Autodesk Fusion 360 part; units mm, degrees
note: some values were not read from the file. Set by a fixed rule: which sketch regions a step uses.
(part 2 of 6)
sketch "Sketch7" plane through (0, 0, 5.5) normal (0, 0, 1) x (1, 0, 0)
  arc A0 (7.002, -1.8799) -> (7.2083, -0.7765) centre (0, 0) ccw
  line L0 (7.2083, -0.7765) -> (7.9414, -0.8554)
  line L1 (7.9414, -0.8554) -> (7.9421, -0.8555)
  spline S0 degree 5 poles (7.9421, -0.8555) (7.9422, -0.8555) (7.9424, -0.8555) (7.9426, -0.8555) (7.943, -0.8556) (7.9436, -0.8556) (7.9443, -0.8557) (7.945, -0.8557) (7.9458, -0.8558) (7.9468, -0.8559) (7.9478, -0.8559) (7.9489, -0.856) (7.9501, -0.8561) (7.9513, -0.8562) (7.9527, -0.8562) (7.9541, -0.8563) (7.9556, -0.8564) (7.9572, -0.8565) (7.9588, -0.8565) (7.9606, -0.8566) (7.9624, -0.8567) (7.9643, -0.8567) (7.9662, -0.8568) (7.9683, -0.8569) (7.9704, -0.8569) (7.9726, -0.8569) (7.9748, -0.857) (7.9771, -0.857) (7.9795, -0.857) (7.982, -0.8571) (7.9846, -0.8571) (7.9872, -0.8571) (7.9899, -0.8571) (7.9926, -0.8571) (7.9954, -0.857) (7.9983, -0.857) (8.0013, -0.857) (8.0043, -0.8569) (8.0074, -0.8569) (8.0105, -0.8568) (8.0137, -0.8567) (8.017, -0.8566) (8.0203, -0.8565) (8.0237, -0.8564) (8.0272, -0.8563) (8.0307, -0.8561) (8.0343, -0.856) (8.038, -0.8558) (8.0417, -0.8556) (8.0455, -0.8554) (8.0493, -0.8552) (8.0532, -0.855) (8.0571, -0.8547) (8.0611, -0.8545) (8.0652, -0.8542) (8.0693, -0.8539) (8.0735, -0.8536) (8.0777, -0.8533) (8.082, -0.8529) (8.0863, -0.8526) (8.0907, -0.8522) (8.0952, -0.8518) (8.0997, -0.8514) (8.1043, -0.851) (8.1089, -0.8505) (8.1136, -0.8501) (8.1183, -0.8496) (8.123, -0.8491) (8.1279, -0.8486) (8.1327, -0.848) (8.1377, -0.8475) (8.1427, -0.8469) (8.1477, -0.8463) (8.1528, -0.8457) (8.1579, -0.845) (8.1631, -0.8444) (8.1683, -0.8437) (8.1736, -0.843) (8.1789, -0.8422) (8.1842, -0.8415) (8.1897, -0.8407) (8.1951, -0.8399) (8.2006, -0.8391) (8.2062, -0.8383) (8.2118, -0.8374) (8.2174, -0.8365) (8.2231, -0.8356) (8.2289, -0.8347) (8.2346, -0.8338) (8.2405, -0.8328) (8.2463, -0.8318) (8.2523, -0.8308) (8.2582, -0.8297) (8.2642, -0.8287) (8.2703, -0.8276) (8.2763, -0.8264) (8.2825, -0.8253) (8.2886, -0.8241) (8.2948, -0.8229) (8.3011, -0.8217) (8.3074, -0.8205) (8.3137, -0.8192) (8.3201, -0.8179) (8.3265, -0.8166) (8.333, -0.8152) (8.3394, -0.8139) (8.346, -0.8125) (8.3525, -0.8111) (8.3591, -0.8096) (8.3658, -0.8081) (8.3725, -0.8066) (8.3792, -0.8051) (8.386, -0.8035) (8.3927, -0.8019) (8.3996, -0.8003) (8.4064, -0.7987) (8.4134, -0.797) (8.4203, -0.7953) (8.4273, -0.7936) (8.4343, -0.7919) (8.4413, -0.7901) (8.4484, -0.7883) (8.4555, -0.7864) (8.4627, -0.7846) (8.4699, -0.7827) (8.4771, -0.7808) (8.4843, -0.7788) (8.4916, -0.7768) (8.4989, -0.7748) (8.5063, -0.7728) (8.5137, -0.7707) (8.5211, -0.7686) (8.5285, -0.7665) (8.536, -0.7643) (8.5435, -0.7622) (8.5511, -0.7599) (8.5586, -0.7577) (8.5662, -0.7554) (8.5739, -0.7531) (8.5815, -0.7508) (8.5892, -0.7484) (8.597, -0.746) (8.6047, -0.7436) (8.6125, -0.7412) (8.6203, -0.7387) (8.6281, -0.7362) (8.636, -0.7336) (8.6439, -0.7311) (8.6518, -0.7284) (8.6598, -0.7258) (8.6678, -0.7231) (8.6758, -0.7204) (8.6838, -0.7177) (8.6919, -0.7149) (8.7, -0.7122) (8.7081, -0.7093) (8.7163, -0.7065) (8.7244, -0.7036) (8.7326, -0.7007) (8.7408, -0.6977) (8.7491, -0.6947) (8.7574, -0.6917) (8.7657, -0.6887) (8.774, -0.6856) (8.7823, -0.6825) (8.7907, -0.6793) (8.7991, -0.6762) (8.8075, -0.673) (8.816, -0.6697) (8.8245, -0.6665) (8.833, -0.6632) (8.8415, -0.6598) (8.85, -0.6565) (8.8586, -0.6531) (8.8672, -0.6496) (8.8758, -0.6462) (8.8844, -0.6427) (8.8931, -0.6391) (8.9017, -0.6356) (8.9104, -0.632) (8.9191, -0.6283) (8.9279, -0.6247) (8.9366, -0.621) (8.9454, -0.6172) (8.9542, -0.6135) (8.963, -0.6097) (8.9719, -0.6058) (8.9808, -0.602) (8.9896, -0.5981) (8.9985, -0.5942) (9.0075, -0.5902) (9.0164, -0.5862) (9.0254, -0.5822) (9.0343, -0.5781) (9.0433, -0.574) (9.0524, -0.5699) (9.0614, -0.5657) (9.0705, -0.5615) (9.0795, -0.5573) (9.0886, -0.553) (9.0977, -0.5487) (9.1069, -0.5444) (9.116, -0.54) (9.1252, -0.5356) (9.1343, -0.5312) (9.1435, -0.5267) (9.1527, -0.5222) (9.162, -0.5176) (9.1712, -0.5131) (9.1805, -0.5085) (9.1898, -0.5038) (9.199, -0.4991) (9.2084, -0.4944) (9.2177, -0.4897) (9.227, -0.4849) (9.2364, -0.4801) (9.2457, -0.4752) (9.2551, -0.4704) (9.2645, -0.4654) (9.2739, -0.4605) (9.2834, -0.4555) (9.2928, -0.4505) (9.3023, -0.4454) (9.3117, -0.4403) (9.3212, -0.4352) (9.3307, -0.43) (9.3402, -0.4249) (9.3497, -0.4196) (9.3593, -0.4144) (9.3688, -0.4091) (9.3784, -0.4037) (9.3879, -0.3984) (9.3975, -0.3929) (9.4071, -0.3875) (9.4167, -0.382) (9.4264, -0.3765) (9.436, -0.371) (9.4456, -0.3654) (9.4553, -0.3598) (9.465, -0.3541) (9.4746, -0.3485) (9.4824, -0.3439) (9.4882, -0.3404) (9.4921, -0.3381) (9.494, -0.337) knots 0 0 0 0 0 0 0.00416667 0.00833333 0.0125 0.01666667 0.02083333 0.025 0.02916667 0.03333333 0.0375 0.04166667 0.04583333 0.05 0.05416667 0.05833333 0.0625 0.06666667 0.07083333 0.075 0.07916667 0.08333333 0.0875 0.09166667 0.09583333 0.1 0.10416667 0.10833333 0.1125 0.11666667 0.12083333 0.125 0.12916667 0.13333333 0.1375 0.14166667 0.14583333 0.15 0.15416667 0.15833333 0.1625 0.16666667 0.17083333 0.175 0.17916667 0.18333333 0.1875 0.19166667 0.19583333 0.2 0.20416667 0.20833333 0.2125 0.21666667 0.22083333 0.225 0.22916667 0.23333333 0.2375 0.24166667 0.24583333 0.25 0.25416667 0.25833333 0.2625 0.26666667 0.27083333 0.275 0.27916667 0.28333333 0.2875 0.29166667 0.29583333 0.3 0.30416667 0.30833333 0.3125 0.31666667 0.32083333 0.325 0.32916667 0.33333333 0.3375 0.34166667 0.34583333 0.35 0.35416667 0.35833333 0.3625 0.36666667 0.37083333 0.375 0.37916667 0.38333333 0.3875 0.39166667 0.39583333 0.4 0.40416667 0.40833333 0.4125 0.41666667 0.42083333 0.425 0.42916667 0.43333333 0.4375 0.44166667 0.44583333 0.45 0.45416667 0.45833333 0.4625 0.46666667 0.47083333 0.475 0.47916667 0.48333333 0.4875 0.49166667 0.49583333 0.5 0.50416667 0.50833333 0.5125 0.51666667 0.52083333 0.525 0.52916667 0.53333333 0.5375 0.54166667 0.54583333 0.55 0.55416667 0.55833333 0.5625 0.56666667 0.57083333 0.575 0.57916667 0.58333333 0.5875 0.59166667 0.59583333 0.6 0.60416667 0.60833333 0.6125 0.61666667 0.62083333 0.625 0.62916667 0.63333333 0.6375 0.64166667 0.64583333 0.65 0.65416667 0.65833333 0.6625 0.66666667 0.67083333 0.675 0.67916667 0.68333333 0.6875 0.69166667 0.69583333 0.7 0.70416667 0.70833333 0.7125 0.71666667 0.72083333 0.725 0.72916667 0.73333333 0.7375 0.74166667 0.74583333 0.75 0.75416667 0.75833333 0.7625 0.76666667 0.77083333 0.775 0.77916667 0.78333333 0.7875 0.79166667 0.79583333 0.8 0.80416667 0.80833333 0.8125 0.81666667 0.82083333 0.825 0.82916667 0.83333333 0.8375 0.84166667 0.84583333 0.85 0.85416667 0.85833333 0.8625 0.86666667 0.87083333 0.875 0.87916667 0.88333333 0.8875 0.89166667 0.89583333 0.9 0.90416667 0.90833333 0.9125 0.91666667 0.92083333 0.925 0.92916667 0.93333333 0.9375 0.94166667 0.94583333 0.95 0.95416667 0.95833333 0.9625 0.96666667 0.97083333 0.975 0.97916667 0.98333333 0.9875 0.99166667 0.99583333 1 1 1 1 1 1
  arc A1 (9.494, -0.337) -> (9.494, 0.337) centre (0, 0) ccw
  spline S1 degree 5 poles (9.494, 0.337) (9.4921, 0.3381) (9.4882, 0.3404) (9.4824, 0.3439) (9.4746, 0.3485) (9.465, 0.3541) (9.4553, 0.3598) (9.4456, 0.3654) (9.436, 0.371) (9.4264, 0.3765) (9.4167, 0.382) (9.4071, 0.3875) (9.3975, 0.3929) (9.3879, 0.3984) (9.3784, 0.4037) (9.3688, 0.4091) (9.3593, 0.4144) (9.3497, 0.4196) (9.3402, 0.4249) (9.3307, 0.43) (9.3212, 0.4352) (9.3117, 0.4403) (9.3023, 0.4454) (9.2928, 0.4505) (9.2834, 0.4555) (9.2739, 0.4605) (9.2645, 0.4654) (9.2551, 0.4704) (9.2457, 0.4752) (9.2364, 0.4801) (9.227, 0.4849) (9.2177, 0.4897) (9.2084, 0.4944) (9.199, 0.4991) (9.1898, 0.5038) (9.1805, 0.5085) (9.1712, 0.5131) (9.162, 0.5176) (9.1527, 0.5222) (9.1435, 0.5267) (9.1343, 0.5312) (9.1252, 0.5356) (9.116, 0.54) (9.1069, 0.5444) (9.0977, 0.5487) (9.0886, 0.553) (9.0795, 0.5573) (9.0705, 0.5615) (9.0614, 0.5657) (9.0524, 0.5699) (9.0433, 0.574) (9.0343, 0.5781) (9.0254, 0.5822) (9.0164, 0.5862) (9.0075, 0.5902) (8.9985, 0.5942) (8.9896, 0.5981) (8.9808, 0.602) (8.9719, 0.6058) (8.963, 0.6097) (8.9542, 0.6135) (8.9454, 0.6172) (8.9366, 0.621) (8.9279, 0.6247) (8.9191, 0.6283) (8.9104, 0.632) (8.9017, 0.6356) (8.8931, 0.6391) (8.8844, 0.6427) (8.8758, 0.6462) (8.8672, 0.6496) (8.8586, 0.6531) (8.85, 0.6565) (8.8415, 0.6598) (8.833, 0.6632) (8.8245, 0.6665) (8.816, 0.6697) (8.8075, 0.673) (8.7991, 0.6762) (8.7907, 0.6793) (8.7823, 0.6825) (8.774, 0.6856) (8.7657, 0.6887) (8.7574, 0.6917) (8.7491, 0.6947) (8.7408, 0.6977) (8.7326, 0.7007) (8.7244, 0.7036) (8.7163, 0.7065) (8.7081, 0.7093) (8.7, 0.7122) (8.6919, 0.7149) (8.6838, 0.7177) (8.6758, 0.7204) (8.6678, 0.7231) (8.6598, 0.7258) (8.6518, 0.7284) (8.6439, 0.7311) (8.636, 0.7336) (8.6281, 0.7362) (8.6203, 0.7387) (8.6125, 0.7412) (8.6047, 0.7436) (8.597, 0.746) (8.5892, 0.7484) (8.5815, 0.7508) (8.5739, 0.7531) (8.5662, 0.7554) (8.5586, 0.7577) (8.5511, 0.7599) (8.5435, 0.7622) (8.536, 0.7643) (8.5285, 0.7665) (8.5211, 0.7686) (8.5137, 0.7707) (8.5063, 0.7728) (8.4989, 0.7748) (8.4916, 0.7768) (8.4843, 0.7788) (8.4771, 0.7808) (8.4699, 0.7827) (8.4627, 0.7846) (8.4555, 0.7864) (8.4484, 0.7883) (8.4413, 0.7901) (8.4343, 0.7919) (8.4273, 0.7936) (8.4203, 0.7953) (8.4134, 0.797) (8.4064, 0.7987) (8.3996, 0.8003) (8.3927, 0.8019) (8.386, 0.8035) (8.3792, 0.8051) (8.3725, 0.8066) (8.3658, 0.8081) (8.3591, 0.8096) (8.3525, 0.8111) (8.346, 0.8125) (8.3394, 0.8139) (8.333, 0.8152) (8.3265, 0.8166) (8.3201, 0.8179) (8.3137, 0.8192) (8.3074, 0.8205) (8.3011, 0.8217) (8.2948, 0.8229) (8.2886, 0.8241) (8.2825, 0.8253) (8.2763, 0.8264) (8.2703, 0.8276) (8.2642, 0.8287) (8.2582, 0.8297) (8.2523, 0.8308) (8.2463, 0.8318) (8.2405, 0.8328) (8.2346, 0.8338) (8.2289, 0.8347) (8.2231, 0.8356) (8.2174, 0.8365) (8.2118, 0.8374) (8.2062, 0.8383) (8.2006, 0.8391) (8.1951, 0.8399) (8.1897, 0.8407) (8.1842, 0.8415) (8.1789, 0.8422) (8.1736, 0.843) (8.1683, 0.8437) (8.1631, 0.8444) (8.1579, 0.845) (8.1528, 0.8457) (8.1477, 0.8463) (8.1427, 0.8469) (8.1377, 0.8475) (8.1327, 0.848) (8.1279, 0.8486) (8.123, 0.8491) (8.1183, 0.8496) (8.1136, 0.8501) (8.1089, 0.8505) (8.1043, 0.851) (8.0997, 0.8514) (8.0952, 0.8518) (8.0907, 0.8522) (8.0863, 0.8526) (8.082, 0.8529) (8.0777, 0.8533) (8.0735, 0.8536) (8.0693, 0.8539) (8.0652, 0.8542) (8.0611, 0.8545) (8.0571, 0.8547) (8.0532, 0.855) (8.0493, 0.8552) (8.0455, 0.8554) (8.0417, 0.8556) (8.038, 0.8558) (8.0343, 0.856) (8.0307, 0.8561) (8.0272, 0.8563) (8.0237, 0.8564) (8.0203, 0.8565) (8.017, 0.8566) (8.0137, 0.8567) (8.0105, 0.8568) (8.0074, 0.8569) (8.0043, 0.8569) (8.0013, 0.857) (7.9983, 0.857) (7.9954, 0.857) (7.9926, 0.8571) (7.9899, 0.8571) (7.9872, 0.8571) (7.9846, 0.8571) (7.982, 0.8571) (7.9795, 0.857) (7.9771, 0.857) (7.9748, 0.857) (7.9726, 0.8569) (7.9704, 0.8569) (7.9683, 0.8569) (7.9662, 0.8568) (7.9643, 0.8567) (7.9624, 0.8567) (7.9606, 0.8566) (7.9588, 0.8565) (7.9572, 0.8565) (7.9556, 0.8564) (7.9541, 0.8563) (7.9527, 0.8562) (7.9513, 0.8562) (7.9501, 0.8561) (7.9489, 0.856) (7.9478, 0.8559) (7.9468, 0.8559) (7.9458, 0.8558) (7.945, 0.8557) (7.9443, 0.8557) (7.9436, 0.8556) (7.943, 0.8556) (7.9426, 0.8555) (7.9424, 0.8555) (7.9422, 0.8555) (7.9421, 0.8555) knots -1 -1 -1 -1 -1 -1 -0.99583333 -0.99166667 -0.9875 -0.98333333 -0.97916667 -0.975 -0.97083333 -0.96666667 -0.9625 -0.95833333 -0.95416667 -0.95 -0.94583333 -0.94166667 -0.9375 -0.93333333 -0.92916667 -0.925 -0.92083333 -0.91666667 -0.9125 -0.90833333 -0.90416667 -0.9 -0.89583333 -0.89166667 -0.8875 -0.88333333 -0.87916667 -0.875 -0.87083333 -0.86666667 -0.8625 -0.85833333 -0.85416667 -0.85 -0.84583333 -0.84166667 -0.8375 -0.83333333 -0.82916667 -0.825 -0.82083333 -0.81666667 -0.8125 -0.80833333 -0.80416667 -0.8 -0.79583333 -0.79166667 -0.7875 -0.78333333 -0.77916667 -0.775 -0.77083333 -0.76666667 -0.7625 -0.75833333 -0.75416667 -0.75 -0.74583333 -0.74166667 -0.7375 -0.73333333 -0.72916667 -0.725 -0.72083333 -0.71666667 -0.7125 -0.70833333 -0.70416667 -0.7 -0.69583333 -0.69166667 -0.6875 -0.68333333 -0.67916667 -0.675 -0.67083333 -0.66666667 -0.6625 -0.65833333 -0.65416667 -0.65 -0.64583333 -0.64166667 -0.6375 -0.63333333 -0.62916667 -0.625 -0.62083333 -0.61666667 -0.6125 -0.60833333 -0.60416667 -0.6 -0.59583333 -0.59166667 -0.5875 -0.58333333 -0.57916667 -0.575 -0.57083333 -0.56666667 -0.5625 -0.55833333 -0.55416667 -0.55 -0.54583333 -0.54166667 -0.5375 -0.53333333 -0.52916667 -0.525 -0.52083333 -0.51666667 -0.5125 -0.50833333 -0.50416667 -0.5 -0.49583333 -0.49166667 -0.4875 -0.48333333 -0.47916667 -0.475 -0.47083333 -0.46666667 -0.4625 -0.45833333 -0.45416667 -0.45 -0.44583333 -0.44166667 -0.4375 -0.43333333 -0.42916667 -0.425 -0.42083333 -0.41666667 -0.4125 -0.40833333 -0.40416667 -0.4 -0.39583333 -0.39166667 -0.3875 -0.38333333 -0.37916667 -0.375 -0.37083333 -0.36666667 -0.3625 -0.35833333 -0.35416667 -0.35 -0.34583333 -0.34166667 -0.3375 -0.33333333 -0.32916667 -0.325 -0.32083333 -0.31666667 -0.3125 -0.30833333 -0.30416667 -0.3 -0.29583333 -0.29166667 -0.2875 -0.28333333 -0.27916667 -0.275 -0.27083333 -0.26666667 -0.2625 -0.25833333 -0.25416667 -0.25 -0.24583333 -0.24166667 -0.2375 -0.23333333 -0.22916667 -0.225 -0.22083333 -0.21666667 -0.2125 -0.20833333 -0.20416667 -0.2 -0.19583333 -0.19166667 -0.1875 -0.18333333 -0.17916667 -0.175 -0.17083333 -0.16666667 -0.1625 -0.15833333 -0.15416667 -0.15 -0.14583333 -0.14166667 -0.1375 -0.13333333 -0.12916667 -0.125 -0.12083333 -0.11666667 -0.1125 -0.10833333 -0.10416667 -0.1 -0.09583333 -0.09166667 -0.0875 -0.08333333 -0.07916667 -0.075 -0.07083333 -0.06666667 -0.0625 -0.05833333 -0.05416667 -0.05 -0.04583333 -0.04166667 -0.0375 -0.03333333 -0.02916667 -0.025 -0.02083333 -0.01666667 -0.0125 -0.00833333 -0.00416667 0 0 0 0 0 0
  line L2 (7.9421, 0.8555) -> (7.9414, 0.8554)
  line L3 (7.9414, 0.8554) -> (7.2083, 0.7765)
  arc A2 (7.2083, 0.7765) -> (7.002, 1.8799) centre (0, 0) ccw
  line L4 (7.002, 1.8799) -> (7.7142, 2.0711)
  line L5 (7.7142, 2.0711) -> (7.7149, 2.0713)
  spline S2 degree 5 poles (7.7149, 2.0713) (7.7149, 2.0713) (7.7151, 2.0714) (7.7153, 2.0714) (7.7157, 2.0715) (7.7163, 2.0717) (7.7169, 2.0719) (7.7176, 2.0721) (7.7184, 2.0723) (7.7193, 2.0726) (7.7203, 2.0729) (7.7213, 2.0732) (7.7225, 2.0736) (7.7237, 2.074) (7.7249, 2.0744) (7.7263, 2.0749) (7.7277, 2.0753) (7.7292, 2.0758) (7.7308, 2.0764) (7.7324, 2.0769) (7.7342, 2.0775) (7.7359, 2.0781) (7.7378, 2.0788) (7.7397, 2.0795) (7.7417, 2.0802) (7.7438, 2.0809) (7.7459, 2.0817) (7.7481, 2.0825) (7.7503, 2.0834) (7.7526, 2.0842) (7.755, 2.0852) (7.7574, 2.0861) (7.7599, 2.0871) (7.7625, 2.0881) (7.7651, 2.0891) (7.7678, 2.0902) (7.7705, 2.0913) (7.7733, 2.0924) (7.7762, 2.0936) (7.7791, 2.0948) (7.7821, 2.096) (7.7851, 2.0973) (7.7882, 2.0986) (7.7913, 2.0999) (7.7945, 2.1013) (7.7977, 2.1027) (7.801, 2.1042) (7.8043, 2.1057) (7.8077, 2.1072) (7.8112, 2.1087) (7.8147, 2.1103) (7.8182, 2.1119) (7.8218, 2.1136) (7.8254, 2.1153) (7.8291, 2.117) (7.8329, 2.1187) (7.8367, 2.1205) (7.8405, 2.1224) (7.8444, 2.1242) (7.8483, 2.1261) (7.8522, 2.1281) (7.8563, 2.13) (7.8603, 2.132) (7.8644, 2.1341) (7.8686, 2.1362) (7.8727, 2.1383) (7.877, 2.1404) (7.8812, 2.1426) (7.8856, 2.1449) (7.8899, 2.1471) (7.8943, 2.1494) (7.8987, 2.1518) (7.9032, 2.1541) (7.9077, 2.1566) (7.9123, 2.159) (7.9168, 2.1615) (7.9215, 2.164) (7.9261, 2.1666) (7.9308, 2.1692) (7.9356, 2.1718) (7.9403, 2.1745) (7.9451, 2.1772) (7.95, 2.18) (7.9549, 2.1827) (7.9598, 2.1856) (7.9647, 2.1884) (7.9697, 2.1913) (7.9747, 2.1943) (7.9798, 2.1972) (7.9849, 2.2002) (7.99, 2.2033) (7.9951, 2.2064) (8.0003, 2.2095) (8.0055, 2.2127) (8.0107, 2.2159) (8.016, 2.2191) (8.0213, 2.2224) (8.0266, 2.2257) (8.032, 2.2291) (8.0374, 2.2325) (8.0428, 2.2359) (8.0482, 2.2394) (8.0537, 2.2429) (8.0592, 2.2464) (8.0647, 2.25) (8.0703, 2.2536) (8.0759, 2.2573) (8.0815, 2.261) (8.0871, 2.2647) (8.0928, 2.2685) (8.0985, 2.2723) (8.1042, 2.2762) (8.1099, 2.2801) (8.1157, 2.284) (8.1215, 2.288) (8.1273, 2.292) (8.1331, 2.2961) (8.139, 2.3001) (8.1449, 2.3043) (8.1508, 2.3084) (8.1567, 2.3126) (8.1627, 2.3169) (8.1686, 2.3212) (8.1746, 2.3255) (8.1806, 2.3298) (8.1867, 2.3342) (8.1927, 2.3387) (8.1988, 2.3432) (8.2049, 2.3477) (8.211, 2.3522) (8.2172, 2.3568) (8.2233, 2.3614) (8.2295, 2.3661) (8.2357, 2.3708) (8.2419, 2.3756) (8.2481, 2.3804) (8.2544, 2.3852) (8.2607, 2.3901) (8.267, 2.395) (8.2733, 2.3999) (8.2796, 2.4049) (8.2859, 2.4099) (8.2923, 2.415) (8.2986, 2.4201) (8.305, 2.4252) (8.3114, 2.4304) (8.3179, 2.4356) (8.3243, 2.4409) (8.3307, 2.4462) (8.3372, 2.4515) (8.3437, 2.4569) (8.3502, 2.4623) (8.3567, 2.4677) (8.3632, 2.4732) (8.3698, 2.4787) (8.3763, 2.4843) (8.3829, 2.4899) (8.3895, 2.4955) (8.396, 2.5012) (8.4026, 2.507) (8.4093, 2.5127) (8.4159, 2.5185) (8.4225, 2.5244) (8.4292, 2.5302) (8.4358, 2.5361) (8.4425, 2.5421) (8.4492, 2.5481) (8.4559, 2.5541) (8.4626, 2.5602) (8.4693, 2.5663) (8.476, 2.5725) (8.4828, 2.5786) (8.4895, 2.5849) (8.4963, 2.5911) (8.503, 2.5974) (8.5098, 2.6038) (8.5166, 2.6102) (8.5234, 2.6166) (8.5302, 2.623) (8.537, 2.6295) (8.5438, 2.6361) (8.5507, 2.6426) (8.5575, 2.6493) (8.5643, 2.6559) (8.5712, 2.6626) (8.578, 2.6693) (8.5849, 2.6761) (8.5918, 2.6829) (8.5986, 2.6897) (8.6055, 2.6966) (8.6124, 2.7035) (8.6193, 2.7105) (8.6262, 2.7175) (8.6331, 2.7245) (8.64, 2.7316) (8.6469, 2.7387) (8.6539, 2.7459) (8.6608, 2.753) (8.6677, 2.7603) (8.6747, 2.7675) (8.6816, 2.7748) (8.6885, 2.7822) (8.6955, 2.7895) (8.7024, 2.797) (8.7094, 2.8044) (8.7164, 2.8119) (8.7233, 2.8194) (8.7303, 2.827) (8.7372, 2.8346) (8.7442, 2.8422) (8.7512, 2.8499) (8.7582, 2.8576) (8.7651, 2.8654) (8.7721, 2.8732) (8.7791, 2.881) (8.7861, 2.8889) (8.7931, 2.8968) (8.8001, 2.9047) (8.807, 2.9127) (8.814, 2.9207) (8.821, 2.9288) (8.828, 2.9369) (8.835, 2.945) (8.842, 2.9532) (8.849, 2.9614) (8.856, 2.9696) (8.863, 2.9779) (8.8699, 2.9862) (8.8769, 2.9946) (8.8839, 3.003) (8.8909, 3.0114) (8.8979, 3.0199) (8.9049, 3.0284) (8.9119, 3.0369) (8.9189, 3.0455) (8.9258, 3.0541) (8.9328, 3.0627) (8.9398, 3.0714) (8.9468, 3.0802) (8.9537, 3.0889) (8.9607, 3.0977) (8.9663, 3.1048) (8.9705, 3.1101) (8.9732, 3.1136) (8.9746, 3.1154) knots 0 0 0 0 0 0 0.00416667 0.00833333 0.0125 0.01666667 0.02083333 0.025 0.02916667 0.03333333 0.0375 0.04166667 0.04583333 0.05 0.05416667 0.05833333 0.0625 0.06666667 0.07083333 0.075 0.07916667 0.08333333 0.0875 0.09166667 0.09583333 0.1 0.10416667 0.10833333 0.1125 0.11666667 0.12083333 0.125 0.12916667 0.13333333 0.1375 0.14166667 0.14583333 0.15 0.15416667 0.15833333 0.1625 0.16666667 0.17083333 0.175 0.17916667 0.18333333 0.1875 0.19166667 0.19583333 0.2 0.20416667 0.20833333 0.2125 0.21666667 0.22083333 0.225 0.22916667 0.23333333 0.2375 0.24166667 0.24583333 0.25 0.25416667 0.25833333 0.2625 0.26666667 0.27083333 0.275 0.27916667 0.28333333 0.2875 0.29166667 0.29583333 0.3 0.30416667 0.30833333 0.3125 0.31666667 0.32083333 0.325 0.32916667 0.33333333 0.3375 0.34166667 0.34583333 0.35 0.35416667 0.35833333 0.3625 0.36666667 0.37083333 0.375 0.37916667 0.38333333 0.3875 0.39166667 0.39583333 0.4 0.40416667 0.40833333 0.4125 0.41666667 0.42083333 0.425 0.42916667 0.43333333 0.4375 0.44166667 0.44583333 0.45 0.45416667 0.45833333 0.4625 0.46666667 0.47083333 0.475 0.47916667 0.48333333 0.4875 0.49166667 0.49583333 0.5 0.50416667 0.50833333 0.5125 0.51666667 0.52083333 0.525 0.52916667 0.53333333 0.5375 0.54166667 0.54583333 0.55 0.55416667 0.55833333 0.5625 0.56666667 0.57083333 0.575 0.57916667 0.58333333 0.5875 0.59166667 0.59583333 0.6 0.60416667 0.60833333 0.6125 0.61666667 0.62083333 0.625 0.62916667 0.63333333 0.6375 0.64166667 0.64583333 0.65 0.65416667 0.65833333 0.6625 0.66666667 0.67083333 0.675 0.67916667 0.68333333 0.6875 0.69166667 0.69583333 0.7 0.70416667 0.70833333 0.7125 0.71666667 0.72083333 0.725 0.72916667 0.73333333 0.7375 0.74166667 0.74583333 0.75 0.75416667 0.75833333 0.7625 0.76666667 0.77083333 0.775 0.77916667 0.78333333 0.7875 0.79166667 0.79583333 0.8 0.80416667 0.80833333 0.8125 0.81666667 0.82083333 0.825 0.82916667 0.83333333 0.8375 0.84166667 0.84583333 0.85 0.85416667 0.85833333 0.8625 0.86666667 0.87083333 0.875 0.87916667 0.88333333 0.8875 0.89166667 0.89583333 0.9 0.90416667 0.90833333 0.9125 0.91666667 0.92083333 0.925 0.92916667 0.93333333 0.9375 0.94166667 0.94583333 0.95 0.95416667 0.95833333 0.9625 0.96666667 0.97083333 0.975 0.97916667 0.98333333 0.9875 0.99166667 0.99583333 1 1 1 1 1 1
  arc A3 (8.9746, 3.1154) -> (8.7312, 3.7439) centre (0, 0) ccw
  spline S3 degree 5 poles (8.7312, 3.7439) (8.729, 3.7442) (8.7245, 3.745) (8.7178, 3.7461) (8.709, 3.7476) (8.6979, 3.7494) (8.6868, 3.7511) (8.6758, 3.7529) (8.6648, 3.7546) (8.6538, 3.7563) (8.6428, 3.758) (8.6319, 3.7596) (8.621, 3.7612) (8.6101, 3.7628) (8.5992, 3.7643) (8.5884, 3.7658) (8.5776, 3.7673) (8.5668, 3.7688) (8.556, 3.7702) (8.5453, 3.7716) (8.5345, 3.773) (8.5239, 3.7744) (8.5132, 3.7757) (8.5025, 3.777) (8.4919, 3.7783) (8.4813, 3.7795) (8.4708, 3.7807) (8.4602, 3.7819) (8.4497, 3.7831) (8.4392, 3.7842) (8.4288, 3.7853) (8.4183, 3.7864) (8.4079, 3.7875) (8.3975, 3.7885) (8.3872, 3.7895) (8.3769, 3.7905) (8.3666, 3.7915) (8.3563, 3.7924) (8.346, 3.7933) (8.3358, 3.7941) (8.3256, 3.795) (8.3155, 3.7958) (8.3053, 3.7966) (8.2952, 3.7974) (8.2852, 3.7981) (8.2751, 3.7989) (8.2651, 3.7995) (8.2551, 3.8002) (8.2451, 3.8009) (8.2352, 3.8015) (8.2253, 3.8021) (8.2154, 3.8026) (8.2056, 3.8032) (8.1958, 3.8037) (8.186, 3.8042) (8.1763, 3.8047) (8.1665, 3.8051) (8.1568, 3.8056) (8.1472, 3.806) (8.1376, 3.8063) (8.128, 3.8067) (8.1184, 3.807) (8.1089, 3.8073) (8.0993, 3.8076) (8.0899, 3.8079) (8.0804, 3.8081) (8.071, 3.8083) (8.0616, 3.8085) (8.0523, 3.8087) (8.043, 3.8088) (8.0337, 3.8089) (8.0245, 3.809) (8.0153, 3.8091) (8.0061, 3.8092) (7.9969, 3.8092) (7.9878, 3.8092) (7.9787, 3.8092) (7.9697, 3.8092) (7.9607, 3.8091) (7.9517, 3.809) (7.9428, 3.809) (7.9338, 3.8088) (7.925, 3.8087) (7.9161, 3.8085) (7.9073, 3.8084) (7.8986, 3.8082) (7.8898, 3.8079) (7.8811, 3.8077) (7.8725, 3.8074) (7.8638, 3.8072) (7.8552, 3.8069) (7.8467, 3.8065) (7.8382, 3.8062) (7.8297, 3.8058) (7.8212, 3.8055) (7.8128, 3.8051) (7.8045, 3.8047) (7.7961, 3.8042) (7.7878, 3.8038) (7.7796, 3.8033) (7.7713, 3.8028) (7.7632, 3.8023) (7.755, 3.8018) (7.7469, 3.8012) (7.7388, 3.8007) (7.7308, 3.8001) (7.7228, 3.7995) (7.7149, 3.7989) (7.707, 3.7983) (7.6991, 3.7976) (7.6913, 3.797) (7.6835, 3.7963) (7.6757, 3.7956) (7.668, 3.7949) (7.6603, 3.7942) (7.6527, 3.7934) (7.6451, 3.7927) (7.6376, 3.7919) (7.6301, 3.7911) (7.6226, 3.7903) (7.6152, 3.7895) (7.6078, 3.7887) (7.6004, 3.7878) (7.5931, 3.787) (7.5859, 3.7861) (7.5787, 3.7852) (7.5715, 3.7843) (7.5644, 3.7834) (7.5573, 3.7825) (7.5503, 3.7815) (7.5433, 3.7806) (7.5363, 3.7796) (7.5294, 3.7786) (7.5225, 3.7776) (7.5157, 3.7766) (7.5089, 3.7756) (7.5022, 3.7746) (7.4955, 3.7736) (7.4889, 3.7725) (7.4823, 3.7715) (7.4757, 3.7704) (7.4692, 3.7693) (7.4628, 3.7682) (7.4564, 3.7672) (7.45, 3.766) (7.4437, 3.7649) (7.4374, 3.7638) (7.4312, 3.7627) (7.425, 3.7615) (7.4189, 3.7604) (7.4128, 3.7592) (7.4068, 3.7581) (7.4008, 3.7569) (7.3949, 3.7557) (7.389, 3.7545) (7.3832, 3.7534) (7.3774, 3.7522) (7.3717, 3.751) (7.366, 3.7498) (7.3603, 3.7485) (7.3548, 3.7473) (7.3492, 3.7461) (7.3437, 3.7449) (7.3383, 3.7436) (7.3329, 3.7424) (7.3276, 3.7412) (7.3223, 3.7399) (7.3171, 3.7387) (7.3119, 3.7374) (7.3068, 3.7362) (7.3017, 3.7349) (7.2967, 3.7337) (7.2918, 3.7324) (7.2869, 3.7312) (7.282, 3.7299) (7.2772, 3.7286) (7.2725, 3.7274) (7.2678, 3.7261) (7.2632, 3.7249) (7.2586, 3.7236) (7.2541, 3.7224) (7.2496, 3.7211) (7.2452, 3.7199) (7.2408, 3.7186) (7.2365, 3.7174) (7.2323, 3.7161) (7.2281, 3.7149) (7.224, 3.7137) (7.2199, 3.7124) (7.2159, 3.7112) (7.212, 3.71) (7.2081, 3.7088) (7.2043, 3.7076) (7.2005, 3.7064) (7.1968, 3.7052) (7.1932, 3.704) (7.1896, 3.7028) (7.186, 3.7016) (7.1826, 3.7005) (7.1792, 3.6993) (7.1758, 3.6982) (7.1726, 3.6971) (7.1693, 3.696) (7.1662, 3.6948) (7.1631, 3.6937) (7.1601, 3.6927) (7.1571, 3.6916) (7.1542, 3.6905) (7.1514, 3.6895) (7.1486, 3.6885) (7.1459, 3.6875) (7.1433, 3.6865) (7.1407, 3.6855) (7.1382, 3.6845) (7.1358, 3.6836) (7.1334, 3.6826) (7.1311, 3.6817) (7.1289, 3.6808) (7.1267, 3.6799) (7.1246, 3.6791) (7.1226, 3.6783) (7.1206, 3.6775) (7.1188, 3.6767) (7.117, 3.6759) (7.1152, 3.6752) (7.1136, 3.6744) (7.112, 3.6738) (7.1104, 3.6731) (7.109, 3.6725) (7.1076, 3.6718) (7.1063, 3.6713) (7.1051, 3.6707) (7.104, 3.6702) (7.1029, 3.6697) (7.1019, 3.6692) (7.101, 3.6688) (7.1001, 3.6684) (7.0994, 3.668) (7.0987, 3.6677) (7.0981, 3.6674) (7.0976, 3.6672) (7.0972, 3.667) (7.097, 3.6669) (7.0968, 3.6668) (7.0968, 3.6668) knots -1 -1 -1 -1 -1 -1 -0.99583333 -0.99166667 -0.9875 -0.98333333 -0.97916667 -0.975 -0.97083333 -0.96666667 -0.9625 -0.95833333 -0.95416667 -0.95 -0.94583333 -0.94166667 -0.9375 -0.93333333 -0.92916667 -0.925 -0.92083333 -0.91666667 -0.9125 -0.90833333 -0.90416667 -0.9 -0.89583333 -0.89166667 -0.8875 -0.88333333 -0.87916667 -0.875 -0.87083333 -0.86666667 -0.8625 -0.85833333 -0.85416667 -0.85 -0.84583333 -0.84166667 -0.8375 -0.83333333 -0.82916667 -0.825 -0.82083333 -0.81666667 -0.8125 -0.80833333 -0.80416667 -0.8 -0.79583333 -0.79166667 -0.7875 -0.78333333 -0.77916667 -0.775 -0.77083333 -0.76666667 -0.7625 -0.75833333 -0.75416667 -0.75 -0.74583333 -0.74166667 -0.7375 -0.73333333 -0.72916667 -0.725 -0.72083333 -0.71666667 -0.7125 -0.70833333 -0.70416667 -0.7 -0.69583333 -0.69166667 -0.6875 -0.68333333 -0.67916667 -0.675 -0.67083333 -0.66666667 -0.6625 -0.65833333 -0.65416667 -0.65 -0.64583333 -0.64166667 -0.6375 -0.63333333 -0.62916667 -0.625 -0.62083333 -0.61666667 -0.6125 -0.60833333 -0.60416667 -0.6 -0.59583333 -0.59166667 -0.5875 -0.58333333 -0.57916667 -0.575 -0.57083333 -0.56666667 -0.5625 -0.55833333 -0.55416667 -0.55 -0.54583333 -0.54166667 -0.5375 -0.53333333 -0.52916667 -0.525 -0.52083333 -0.51666667 -0.5125 -0.50833333 -0.50416667 -0.5 -0.49583333 -0.49166667 -0.4875 -0.48333333 -0.47916667 -0.475 -0.47083333 -0.46666667 -0.4625 -0.45833333 -0.45416667 -0.45 -0.44583333 -0.44166667 -0.4375 -0.43333333 -0.42916667 -0.425 -0.42083333 -0.41666667 -0.4125 -0.40833333 -0.40416667 -0.4 -0.39583333 -0.39166667 -0.3875 -0.38333333 -0.37916667 -0.375 -0.37083333 -0.36666667 -0.3625 -0.35833333 -0.35416667 -0.35 -0.34583333 -0.34166667 -0.3375 -0.33333333 -0.32916667 -0.325 -0.32083333 -0.31666667 -0.3125 -0.30833333 -0.30416667 -0.3 -0.29583333 -0.29166667 -0.2875 -0.28333333 -0.27916667 -0.275 -0.27083333 -0.26666667 -0.2625 -0.25833333 -0.25416667 -0.25 -0.24583333 -0.24166667 -0.2375 -0.23333333 -0.22916667 -0.225 -0.22083333 -0.21666667 -0.2125 -0.20833333 -0.20416667 -0.2 -0.19583333 -0.19166667 -0.1875 -0.18333333 -0.17916667 -0.175 -0.17083333 -0.16666667 -0.1625 -0.15833333 -0.15416667 -0.15 -0.14583333 -0.14166667 -0.1375 -0.13333333 -0.12916667 -0.125 -0.12083333 -0.11666667 -0.1125 -0.10833333 -0.10416667 -0.1 -0.09583333 -0.09166667 -0.0875 -0.08333333 -0.07916667 -0.075 -0.07083333 -0.06666667 -0.0625 -0.05833333 -0.05416667 -0.05 -0.04583333 -0.04166667 -0.0375 -0.03333333 -0.02916667 -0.025 -0.02083333 -0.01666667 -0.0125 -0.00833333 -0.00416667 0 0 0 0 0 0
  line L6 (7.0968, 3.6668) -> (7.0962, 3.6665)
  line L7 (7.0962, 3.6665) -> (6.441, 3.328)
  arc A4 (6.441, 3.328) -> (5.8501, 4.2824) centre (0, 0) ccw
  line L8 (5.8501, 4.2824) -> (6.4451, 4.7179)
  line L9 (6.4451, 4.7179) -> (6.4457, 4.7184)
  spline S4 degree 5 poles (6.4457, 4.7184) (6.4457, 4.7184) (6.4458, 4.7185) (6.446, 4.7186) (6.4464, 4.7189) (6.4468, 4.7192) (6.4473, 4.7196) (6.4479, 4.7201) (6.4486, 4.7206) (6.4493, 4.7212) (6.4501, 4.7218) (6.451, 4.7225) (6.4519, 4.7233) (6.4529, 4.7241) (6.4539, 4.7249) (6.455, 4.7258) (6.4562, 4.7268) (6.4574, 4.7278) (6.4587, 4.7288) (6.46, 4.7299) (6.4614, 4.7311) (6.4628, 4.7323) (6.4643, 4.7336) (6.4659, 4.735) (6.4675, 4.7363) (6.4691, 4.7378) (6.4708, 4.7393) (6.4726, 4.7408) (6.4743, 4.7424) (6.4762, 4.7441) (6.4781, 4.7458) (6.48, 4.7475) (6.482, 4.7493) (6.484, 4.7512) (6.4861, 4.7531) (6.4882, 4.7551) (6.4903, 4.7571) (6.4925, 4.7592) (6.4948, 4.7613) (6.4971, 4.7635) (6.4994, 4.7657) (6.5017, 4.768) (6.5041, 4.7703) (6.5066, 4.7727) (6.509, 4.7751) (6.5115, 4.7776) (6.5141, 4.7801) (6.5167, 4.7827) (6.5193, 4.7853) (6.5219, 4.788) (6.5246, 4.7908) (6.5274, 4.7936) (6.5301, 4.7964) (6.5329, 4.7993) (6.5357, 4.8022) (6.5386, 4.8052) (6.5414, 4.8083) (6.5443, 4.8113) (6.5473, 4.8145) (6.5503, 4.8177) (6.5533, 4.8209) (6.5563, 4.8242) (6.5593, 4.8275) (6.5624, 4.8309) (6.5655, 4.8344) (6.5687, 4.8379) (6.5718, 4.8414) (6.575, 4.845) (6.5782, 4.8486) (6.5815, 4.8523) (6.5847, 4.856) (6.588, 4.8598) (6.5913, 4.8636) (6.5947, 4.8675) (6.598, 4.8715) (6.6014, 4.8754) (6.6048, 4.8795) (6.6082, 4.8835) (6.6117, 4.8876) (6.6151, 4.8918) (6.6186, 4.896) (6.6221, 4.9003) (6.6257, 4.9046) (6.6292, 4.909) (6.6328, 4.9134) (6.6363, 4.9178) (6.6399, 4.9223) (6.6436, 4.9269) (6.6472, 4.9315) (6.6508, 4.9361) (6.6545, 4.9408) (6.6582, 4.9456) (6.6619, 4.9503) (6.6656, 4.9552) (6.6693, 4.9601) (6.6731, 4.965) (6.6768, 4.97) (6.6806, 4.975) (6.6844, 4.98) (6.6882, 4.9852) (6.692, 4.9903) (6.6958, 4.9955) (6.6996, 5.0008) (6.7035, 5.0061) (6.7074, 5.0114) (6.7112, 5.0168) (6.7151, 5.0222) (6.719, 5.0277) (6.7229, 5.0332) (6.7268, 5.0388) (6.7308, 5.0444) (6.7347, 5.0501) (6.7386, 5.0558) (6.7426, 5.0615) (6.7465, 5.0673) (6.7505, 5.0731) (6.7545, 5.079) (6.7585, 5.085) (6.7625, 5.0909) (6.7665, 5.097) (6.7705, 5.103) (6.7745, 5.1091) (6.7785, 5.1153) (6.7825, 5.1215) (6.7866, 5.1277) (6.7906, 5.134) (6.7947, 5.1403) (6.7987, 5.1467) (6.8028, 5.1531) (6.8068, 5.1595) (6.8109, 5.1661) (6.815, 5.1726) (6.819, 5.1792) (6.8231, 5.1858) (6.8272, 5.1925) (6.8313, 5.1992) (6.8354, 5.206) (6.8395, 5.2128) (6.8435, 5.2196) (6.8476, 5.2265) (6.8517, 5.2334) (6.8558, 5.2404) (6.8599, 5.2474) (6.864, 5.2545) (6.8681, 5.2616) (6.8722, 5.2687) (6.8763, 5.2759) (6.8804, 5.2831) (6.8845, 5.2904) (6.8886, 5.2977) (6.8927, 5.305) (6.8968, 5.3124) (6.9009, 5.3199) (6.905, 5.3273) (6.9091, 5.3349) (6.9132, 5.3424) (6.9173, 5.35) (6.9214, 5.3576) (6.9255, 5.3653) (6.9296, 5.373) (6.9337, 5.3808) (6.9378, 5.3886) (6.9419, 5.3965) (6.9459, 5.4043) (6.95, 5.4123) (6.9541, 5.4202) (6.9582, 5.4282) (6.9622, 5.4363) (6.9663, 5.4444) (6.9703, 5.4525) (6.9744, 5.4606) (6.9784, 5.4688) (6.9825, 5.4771) (6.9865, 5.4854) (6.9906, 5.4937) (6.9946, 5.5021) (6.9986, 5.5105) (7.0026, 5.5189) (7.0066, 5.5274) (7.0106, 5.5359) (7.0146, 5.5444) (7.0186, 5.553) (7.0226, 5.5617) (7.0266, 5.5704) (7.0305, 5.5791) (7.0345, 5.5878) (7.0385, 5.5966) (7.0424, 5.6054) (7.0464, 5.6143) (7.0503, 5.6232) (7.0542, 5.6321) (7.0581, 5.6411) (7.062, 5.6501) (7.0659, 5.6592) (7.0698, 5.6683) (7.0737, 5.6774) (7.0776, 5.6866) (7.0814, 5.6958) (7.0853, 5.705) (7.0891, 5.7143) (7.093, 5.7236) (7.0968, 5.733) (7.1006, 5.7423) (7.1044, 5.7518) (7.1082, 5.7612) (7.112, 5.7707) (7.1158, 5.7803) (7.1195, 5.7898) (7.1233, 5.7994) (7.127, 5.8091) (7.1307, 5.8188) (7.1344, 5.8285) (7.1382, 5.8382) (7.1418, 5.848) (7.1455, 5.8578) (7.1492, 5.8677) (7.1529, 5.8776) (7.1565, 5.8875) (7.1601, 5.8975) (7.1637, 5.9075) (7.1674, 5.9175) (7.1709, 5.9276) (7.1745, 5.9377) (7.1781, 5.9479) (7.1816, 5.958) (7.1852, 5.9682) (7.1887, 5.9785) (7.1922, 5.9888) (7.1957, 5.9991) (7.1992, 6.0094) (7.2027, 6.0198) (7.2061, 6.0302) (7.2096, 6.0407) (7.213, 6.0512) (7.2164, 6.0617) (7.2198, 6.0722) (7.2232, 6.0828) (7.2266, 6.0934) (7.2299, 6.1041) (7.2333, 6.1148) (7.2366, 6.1255) (7.2392, 6.1341) (7.2412, 6.1406) (7.2425, 6.1449) (7.2432, 6.1471) knots 0 0 0 0 0 0 0.00416667 0.00833333 0.0125 0.01666667 0.02083333 0.025 0.02916667 0.03333333 0.0375 0.04166667 0.04583333 0.05 0.05416667 0.05833333 0.0625 0.06666667 0.07083333 0.075 0.07916667 0.08333333 0.0875 0.09166667 0.09583333 0.1 0.10416667 0.10833333 0.1125 0.11666667 0.12083333 0.125 0.12916667 0.13333333 0.1375 0.14166667 0.14583333 0.15 0.15416667 0.15833333 0.1625 0.16666667 0.17083333 0.175 0.17916667 0.18333333 0.1875 0.19166667 0.19583333 0.2 0.20416667 0.20833333 0.2125 0.21666667 0.22083333 0.225 0.22916667 0.23333333 0.2375 0.24166667 0.24583333 0.25 0.25416667 0.25833333 0.2625 0.26666667 0.27083333 0.275 0.27916667 0.28333333 0.2875 0.29166667 0.29583333 0.3 0.30416667 0.30833333 0.3125 0.31666667 0.32083333 0.325 0.32916667 0.33333333 0.3375 0.34166667 0.34583333 0.35 0.35416667 0.35833333 0.3625 0.36666667 0.37083333 0.375 0.37916667 0.38333333 0.3875 0.39166667 0.39583333 0.4 0.40416667 0.40833333 0.4125 0.41666667 0.42083333 0.425 0.42916667 0.43333333 0.4375 0.44166667 0.44583333 0.45 0.45416667 0.45833333 0.4625 0.46666667 0.47083333 0.475 0.47916667 0.48333333 0.4875 0.49166667 0.49583333 0.5 0.50416667 0.50833333 0.5125 0.51666667 0.52083333 0.525 0.52916667 0.53333333 0.5375 0.54166667 0.54583333 0.55 0.55416667 0.55833333 0.5625 0.56666667 0.57083333 0.575 0.57916667 0.58333333 0.5875 0.59166667 0.59583333 0.6 0.60416667 0.60833333 0.6125 0.61666667 0.62083333 0.625 0.62916667 0.63333333 0.6375 0.64166667 0.64583333 0.65 0.65416667 0.65833333 0.6625 0.66666667 0.67083333 0.675 0.67916667 0.68333333 0.6875 0.69166667 0.69583333 0.7 0.70416667 0.70833333 0.7125 0.71666667 0.72083333 0.725 0.72916667 0.73333333 0.7375 0.74166667 0.74583333 0.75 0.75416667 0.75833333 0.7625 0.76666667 0.77083333 0.775 0.77916667 0.78333333 0.7875 0.79166667 0.79583333 0.8 0.80416667 0.80833333 0.8125 0.81666667 0.82083333 0.825 0.82916667 0.83333333 0.8375 0.84166667 0.84583333 0.85 0.85416667 0.85833333 0.8625 0.86666667 0.87083333 0.875 0.87916667 0.88333333 0.8875 0.89166667 0.89583333 0.9 0.90416667 0.90833333 0.9125 0.91666667 0.92083333 0.925 0.92916667 0.93333333 0.9375 0.94166667 0.94583333 0.95 0.95416667 0.95833333 0.9625 0.96666667 0.97083333 0.975 0.97916667 0.98333333 0.9875 0.99166667 0.99583333 1 1 1 1 1 1
  arc A5 (7.2432, 6.1471) -> (6.7892, 6.6451) centre (0, 0) ccw
  spline S5 degree 5 poles (6.7892, 6.6451) (6.7869, 6.6446) (6.7825, 6.6437) (6.7759, 6.6424) (6.7671, 6.6405) (6.7561, 6.6382) (6.7452, 6.6359) (6.7342, 6.6335) (6.7234, 6.6311) (6.7125, 6.6287) (6.7017, 6.6263) (6.6909, 6.6239) (6.6801, 6.6215) (6.6694, 6.619) (6.6587, 6.6165) (6.6481, 6.614) (6.6374, 6.6115) (6.6268, 6.609) (6.6163, 6.6064) (6.6057, 6.6039) (6.5953, 6.6013) (6.5848, 6.5987) (6.5744, 6.5961) (6.564, 6.5934) (6.5536, 6.5908) (6.5433, 6.5881) (6.533, 6.5854) (6.5227, 6.5827) (6.5125, 6.58) (6.5023, 6.5773) (6.4922, 6.5746) (6.482, 6.5718) (6.472, 6.569) (6.4619, 6.5662) (6.4519, 6.5634) (6.4419, 6.5606) (6.432, 6.5578) (6.422, 6.5549) (6.4122, 6.5521) (6.4023, 6.5492) (6.3925, 6.5463) (6.3827, 6.5434) (6.373, 6.5405) (6.3633, 6.5375) (6.3536, 6.5346) (6.344, 6.5316) (6.3344, 6.5287) (6.3249, 6.5257) (6.3153, 6.5227) (6.3059, 6.5197) (6.2964, 6.5167) (6.287, 6.5136) (6.2776, 6.5106) (6.2683, 6.5075) (6.259, 6.5044) (6.2497, 6.5014) (6.2405, 6.4983) (6.2313, 6.4952) (6.2222, 6.4921) (6.213, 6.4889) (6.204, 6.4858) (6.1949, 6.4826) (6.1859, 6.4795) (6.177, 6.4763) (6.168, 6.4731) (6.1591, 6.4699) (6.1503, 6.4667) (6.1415, 6.4635) (6.1327, 6.4603) (6.124, 6.4571) (6.1153, 6.4538) (6.1066, 6.4506) (6.098, 6.4473) (6.0894, 6.4441) (6.0809, 6.4408) (6.0724, 6.4375) (6.0639, 6.4342) (6.0555, 6.4309) (6.0471, 6.4276) (6.0387, 6.4243) (6.0304, 6.421) (6.0222, 6.4177) (6.014, 6.4143) (6.0058, 6.411) (5.9976, 6.4076) (5.9895, 6.4043) (5.9814, 6.4009) (5.9734, 6.3976) (5.9654, 6.3942) (5.9575, 6.3908) (5.9496, 6.3874) (5.9417, 6.384) (5.9339, 6.3807) (5.9261, 6.3773) (5.9184, 6.3739) (5.9107, 6.3704) (5.903, 6.367) (5.8954, 6.3636) (5.8879, 6.3602) (5.8803, 6.3568) (5.8728, 6.3534) (5.8654, 6.3499) (5.858, 6.3465) (5.8506, 6.3431) (5.8433, 6.3396) (5.836, 6.3362) (5.8288, 6.3327) (5.8216, 6.3293) (5.8144, 6.3259) (5.8073, 6.3224) (5.8003, 6.319) (5.7932, 6.3155) (5.7863, 6.3121) (5.7793, 6.3086) (5.7724, 6.3052) (5.7656, 6.3017) (5.7588, 6.2983) (5.752, 6.2948) (5.7453, 6.2914) (5.7386, 6.288) (5.732, 6.2845) (5.7254, 6.2811) (5.7189, 6.2776) (5.7124, 6.2742) (5.7059, 6.2708) (5.6995, 6.2673) (5.6932, 6.2639) (5.6869, 6.2605) (5.6806, 6.257) (5.6744, 6.2536) (5.6682, 6.2502) (5.6621, 6.2468) (5.656, 6.2434) (5.6499, 6.24) (5.6439, 6.2366) (5.638, 6.2332) (5.6321, 6.2298) (5.6262, 6.2264) (5.6204, 6.2231) (5.6146, 6.2197) (5.6089, 6.2163) (5.6032, 6.213) (5.5976, 6.2097) (5.592, 6.2063) (5.5865, 6.203) (5.581, 6.1997) (5.5756, 6.1964) (5.5702, 6.1931) (5.5648, 6.1898) (5.5595, 6.1865) (5.5543, 6.1832) (5.5491, 6.18) (5.5439, 6.1767) (5.5388, 6.1735) (5.5337, 6.1702) (5.5287, 6.167) (5.5238, 6.1638) (5.5189, 6.1606) (5.514, 6.1574) (5.5092, 6.1543) (5.5044, 6.1511) (5.4997, 6.148) (5.495, 6.1449) (5.4904, 6.1417) (5.4858, 6.1386) (5.4813, 6.1356) (5.4768, 6.1325) (5.4724, 6.1295) (5.4681, 6.1264) (5.4637, 6.1234) (5.4595, 6.1204) (5.4552, 6.1174) (5.4511, 6.1145) (5.447, 6.1115) (5.4429, 6.1086) (5.4389, 6.1057) (5.4349, 6.1028) (5.431, 6.0999) (5.4271, 6.0971) (5.4233, 6.0943) (5.4195, 6.0915) (5.4158, 6.0887) (5.4122, 6.0859) (5.4086, 6.0832) (5.405, 6.0805) (5.4015, 6.0778) (5.3981, 6.0751) (5.3947, 6.0725) (5.3913, 6.0699) (5.388, 6.0673) (5.3848, 6.0647) (5.3816, 6.0622) (5.3785, 6.0597) (5.3754, 6.0572) (5.3724, 6.0548) (5.3694, 6.0523) (5.3665, 6.0499) (5.3636, 6.0476) (5.3608, 6.0453) (5.358, 6.0429) (5.3553, 6.0407) (5.3527, 6.0384) (5.3501, 6.0362) (5.3475, 6.0341) (5.3451, 6.0319) (5.3426, 6.0298) (5.3402, 6.0278) (5.3379, 6.0257) (5.3357, 6.0237) (5.3335, 6.0218) (5.3313, 6.0198) (5.3292, 6.018) (5.3272, 6.0161) (5.3252, 6.0143) (5.3233, 6.0126) (5.3214, 6.0108) (5.3196, 6.0091) (5.3178, 6.0075) (5.3161, 6.0059) (5.3145, 6.0044) (5.3129, 6.0029) (5.3114, 6.0014) (5.3099, 6) (5.3085, 5.9986) (5.3071, 5.9973) (5.3058, 5.996) (5.3046, 5.9948) (5.3034, 5.9936) (5.3023, 5.9925) (5.3012, 5.9915) (5.3002, 5.9904) (5.2993, 5.9895) (5.2984, 5.9886) (5.2976, 5.9877) (5.2968, 5.9869) (5.2961, 5.9862) (5.2955, 5.9855) (5.2949, 5.9849) (5.2944, 5.9844) (5.2939, 5.9839) (5.2935, 5.9835) (5.2933, 5.9832) (5.2931, 5.983) (5.293, 5.9829) (5.293, 5.9828) knots -1 -1 -1 -1 -1 -1 -0.99583333 -0.99166667 -0.9875 -0.98333333 -0.97916667 -0.975 -0.97083333 -0.96666667 -0.9625 -0.95833333 -0.95416667 -0.95 -0.94583333 -0.94166667 -0.9375 -0.93333333 -0.92916667 -0.925 -0.92083333 -0.91666667 -0.9125 -0.90833333 -0.90416667 -0.9 -0.89583333 -0.89166667 -0.8875 -0.88333333 -0.87916667 -0.875 -0.87083333 -0.86666667 -0.8625 -0.85833333 -0.85416667 -0.85 -0.84583333 -0.84166667 -0.8375 -0.83333333 -0.82916667 -0.825 -0.82083333 -0.81666667 -0.8125 -0.80833333 -0.80416667 -0.8 -0.79583333 -0.79166667 -0.7875 -0.78333333 -0.77916667 -0.775 -0.77083333 -0.76666667 -0.7625 -0.75833333 -0.75416667 -0.75 -0.74583333 -0.74166667 -0.7375 -0.73333333 -0.72916667 -0.725 -0.72083333 -0.71666667 -0.7125 -0.70833333 -0.70416667 -0.7 -0.69583333 -0.69166667 -0.6875 -0.68333333 -0.67916667 -0.675 -0.67083333 -0.66666667 -0.6625 -0.65833333 -0.65416667 -0.65 -0.64583333 -0.64166667 -0.6375 -0.63333333 -0.62916667 -0.625 -0.62083333 -0.61666667 -0.6125 -0.60833333 -0.60416667 -0.6 -0.59583333 -0.59166667 -0.5875 -0.58333333 -0.57916667 -0.575 -0.57083333 -0.56666667 -0.5625 -0.55833333 -0.55416667 -0.55 -0.54583333 -0.54166667 -0.5375 -0.53333333 -0.52916667 -0.525 -0.52083333 -0.51666667 -0.5125 -0.50833333 -0.50416667 -0.5 -0.49583333 -0.49166667 -0.4875 -0.48333333 -0.47916667 -0.475 -0.47083333 -0.46666667 -0.4625 -0.45833333 -0.45416667 -0.45 -0.44583333 -0.44166667 -0.4375 -0.43333333 -0.42916667 -0.425 -0.42083333 -0.41666667 -0.4125 -0.40833333 -0.40416667 -0.4 -0.39583333 -0.39166667 -0.3875 -0.38333333 -0.37916667 -0.375 -0.37083333 -0.36666667 -0.3625 -0.35833333 -0.35416667 -0.35 -0.34583333 -0.34166667 -0.3375 -0.33333333 -0.32916667 -0.325 -0.32083333 -0.31666667 -0.3125 -0.30833333 -0.30416667 -0.3 -0.29583333 -0.29166667 -0.2875 -0.28333333 -0.27916667 -0.275 -0.27083333 -0.26666667 -0.2625 -0.25833333 -0.25416667 -0.25 -0.24583333 -0.24166667 -0.2375 -0.23333333 -0.22916667 -0.225 -0.22083333 -0.21666667 -0.2125 -0.20833333 -0.20416667 -0.2 -0.19583333 -0.19166667 -0.1875 -0.18333333 -0.17916667 -0.175 -0.17083333 -0.16666667 -0.1625 -0.15833333 -0.15416667 -0.15 -0.14583333 -0.14166667 -0.1375 -0.13333333 -0.12916667 -0.125 -0.12083333 -0.11666667 -0.1125 -0.10833333 -0.10416667 -0.1 -0.09583333 -0.09166667 -0.0875 -0.08333333 -0.07916667 -0.075 -0.07083333 -0.06666667 -0.0625 -0.05833333 -0.05416667 -0.05 -0.04583333 -0.04166667 -0.0375 -0.03333333 -0.02916667 -0.025 -0.02083333 -0.01666667 -0.0125 -0.00833333 -0.00416667 0 0 0 0 0 0
  line L10 (5.293, 5.9828) -> (5.2925, 5.9823)
  line L11 (5.2925, 5.9823) -> (4.8039, 5.43)
  arc A6 (4.8039, 5.43) -> (3.9081, 6.1065) centre (0, 0) ccw
  line L12 (3.9081, 6.1065) -> (4.3056, 6.7276)
  line L13 (4.3056, 6.7276) -> (4.3059, 6.7282)
  spline S6 degree 5 poles (4.3059, 6.7282) (4.306, 6.7282) (4.306, 6.7284) (4.3062, 6.7286) (4.3064, 6.7289) (4.3067, 6.7294) (4.307, 6.73) (4.3074, 6.7306) (4.3079, 6.7314) (4.3083, 6.7322) (4.3088, 6.733) (4.3094, 6.734) (4.31, 6.735) (4.3106, 6.7361) (4.3113, 6.7373) (4.312, 6.7385) (4.3127, 6.7398) (4.3135, 6.7412) (4.3143, 6.7426) (4.3151, 6.7442) (4.316, 6.7458) (4.3169, 6.7474) (4.3178, 6.7492) (4.3188, 6.751) (4.3198, 6.7528) (4.3208, 6.7548) (4.3218, 6.7568) (4.3229, 6.7588) (4.324, 6.761) (4.3251, 6.7632) (4.3262, 6.7655) (4.3274, 6.7678) (4.3286, 6.7702) (4.3298, 6.7727) (4.3311, 6.7752) (4.3323, 6.7778) (4.3336, 6.7804) (4.3349, 6.7832) (4.3362, 6.786) (4.3376, 6.7888) (4.3389, 6.7917) (4.3403, 6.7947) (4.3417, 6.7977) (4.3431, 6.8008) (4.3445, 6.804) (4.346, 6.8072) (4.3474, 6.8105) (4.3489, 6.8138) (4.3504, 6.8172) (4.3519, 6.8207) (4.3534, 6.8242) (4.3549, 6.8278) (4.3565, 6.8315) (4.358, 6.8352) (4.3596, 6.8389) (4.3612, 6.8427) (4.3628, 6.8466) (4.3644, 6.8505) (4.366, 6.8545) (4.3676, 6.8586) (4.3692, 6.8627) (4.3709, 6.8668) (4.3725, 6.8711) (4.3741, 6.8753) (4.3758, 6.8797) (4.3775, 6.8841) (4.3791, 6.8885) (4.3808, 6.893) (4.3825, 6.8975) (4.3842, 6.9021) (4.3859, 6.9068) (4.3876, 6.9115) (4.3893, 6.9163) (4.391, 6.9211) (4.3927, 6.926) (4.3944, 6.9309) (4.3961, 6.9359) (4.3979, 6.9409) (4.3996, 6.946) (4.4013, 6.9511) (4.403, 6.9563) (4.4048, 6.9616) (4.4065, 6.9669) (4.4082, 6.9722) (4.4099, 6.9776) (4.4117, 6.9831) (4.4134, 6.9886) (4.4151, 6.9941) (4.4169, 6.9997) (4.4186, 7.0054) (4.4203, 7.0111) (4.422, 7.0168) (4.4237, 7.0226) (4.4255, 7.0285) (4.4272, 7.0344) (4.4289, 7.0403) (4.4306, 7.0463) (4.4323, 7.0523) (4.434, 7.0584) (4.4357, 7.0646) (4.4374, 7.0707) (4.4391, 7.077) (4.4408, 7.0833) (4.4424, 7.0896) (4.4441, 7.096) (4.4458, 7.1024) (4.4474, 7.1089) (4.4491, 7.1154) (4.4507, 7.1219) (4.4524, 7.1285) (4.454, 7.1352) (4.4556, 7.1419) (4.4572, 7.1486) (4.4588, 7.1554) (4.4604, 7.1623) (4.462, 7.1691) (4.4636, 7.1761) (4.4652, 7.183) (4.4668, 7.19) (4.4683, 7.1971) (4.4699, 7.2042) (4.4714, 7.2113) (4.4729, 7.2185) (4.4745, 7.2258) (4.476, 7.233) (4.4775, 7.2404) (4.4789, 7.2477) (4.4804, 7.2551) (4.4819, 7.2626) (4.4833, 7.27) (4.4848, 7.2776) (4.4862, 7.2852) (4.4876, 7.2928) (4.489, 7.3004) (4.4904, 7.3081) (4.4918, 7.3159) (4.4932, 7.3236) (4.4945, 7.3315) (4.4959, 7.3393) (4.4972, 7.3472) (4.4985, 7.3552) (4.4998, 7.3631) (4.5011, 7.3712) (4.5024, 7.3792) (4.5036, 7.3873) (4.5049, 7.3955) (4.5061, 7.4036) (4.5073, 7.4119) (4.5085, 7.4201) (4.5097, 7.4284) (4.5109, 7.4367) (4.512, 7.4451) (4.5132, 7.4535) (4.5143, 7.462) (4.5154, 7.4705) (4.5165, 7.479) (4.5176, 7.4876) (4.5186, 7.4962) (4.5197, 7.5048) (4.5207, 7.5135) (4.5217, 7.5222) (4.5227, 7.531) (4.5237, 7.5397) (4.5246, 7.5486) (4.5256, 7.5574) (4.5265, 7.5663) (4.5274, 7.5753) (4.5283, 7.5842) (4.5291, 7.5932) (4.53, 7.6023) (4.5308, 7.6113) (4.5316, 7.6205) (4.5324, 7.6296) (4.5332, 7.6388) (4.5339, 7.648) (4.5347, 7.6572) (4.5354, 7.6665) (4.5361, 7.6759) (4.5368, 7.6852) (4.5374, 7.6946) (4.5381, 7.704) (4.5387, 7.7135) (4.5393, 7.723) (4.5398, 7.7325) (4.5404, 7.742) (4.5409, 7.7516) (4.5414, 7.7613) (4.5419, 7.7709) (4.5424, 7.7806) (4.5429, 7.7903) (4.5433, 7.8001) (4.5437, 7.8099) (4.5441, 7.8197) (4.5445, 7.8295) (4.5448, 7.8394) (4.5451, 7.8493) (4.5454, 7.8593) (4.5457, 7.8693) (4.5459, 7.8793) (4.5462, 7.8893) (4.5464, 7.8994) (4.5466, 7.9095) (4.5467, 7.9196) (4.5469, 7.9298) (4.547, 7.94) (4.5471, 7.9502) (4.5472, 7.9604) (4.5472, 7.9707) (4.5472, 7.981) (4.5472, 7.9914) (4.5472, 8.0018) (4.5472, 8.0122) (4.5471, 8.0226) (4.547, 8.0331) (4.5469, 8.0435) (4.5468, 8.0541) (4.5466, 8.0646) (4.5464, 8.0752) (4.5462, 8.0858) (4.546, 8.0964) (4.5457, 8.1071) (4.5454, 8.1178) (4.5451, 8.1285) (4.5448, 8.1392) (4.5444, 8.15) (4.544, 8.1608) (4.5436, 8.1716) (4.5432, 8.1825) (4.5427, 8.1934) (4.5422, 8.2043) (4.5417, 8.2152) (4.5412, 8.2262) (4.5406, 8.2372) (4.54, 8.2482) (4.5394, 8.2592) (4.5387, 8.2703) (4.5381, 8.2814) (4.5374, 8.2925) (4.5367, 8.3037) (4.5359, 8.3148) (4.5351, 8.326) (4.5345, 8.335) (4.534, 8.3417) (4.5337, 8.3462) (4.5335, 8.3485) knots 0 0 0 0 0 0 0.00416667 0.00833333 0.0125 0.01666667 0.02083333 0.025 0.02916667 0.03333333 0.0375 0.04166667 0.04583333 0.05 0.05416667 0.05833333 0.0625 0.06666667 0.07083333 0.075 0.07916667 0.08333333 0.0875 0.09166667 0.09583333 0.1 0.10416667 0.10833333 0.1125 0.11666667 0.12083333 0.125 0.12916667 0.13333333 0.1375 0.14166667 0.14583333 0.15 0.15416667 0.15833333 0.1625 0.16666667 0.17083333 0.175 0.17916667 0.18333333 0.1875 0.19166667 0.19583333 0.2 0.20416667 0.20833333 0.2125 0.21666667 0.22083333 0.225 0.22916667 0.23333333 0.2375 0.24166667 0.24583333 0.25 0.25416667 0.25833333 0.2625 0.26666667 0.27083333 0.275 0.27916667 0.28333333 0.2875 0.29166667 0.29583333 0.3 0.30416667 0.30833333 0.3125 0.31666667 0.32083333 0.325 0.32916667 0.33333333 0.3375 0.34166667 0.34583333 0.35 0.35416667 0.35833333 0.3625 0.36666667 0.37083333 0.375 0.37916667 0.38333333 0.3875 0.39166667 0.39583333 0.4 0.40416667 0.40833333 0.4125 0.41666667 0.42083333 0.425 0.42916667 0.43333333 0.4375 0.44166667 0.44583333 0.45 0.45416667 0.45833333 0.4625 0.46666667 0.47083333 0.475 0.47916667 0.48333333 0.4875 0.49166667 0.49583333 0.5 0.50416667 0.50833333 0.5125 0.51666667 0.52083333 0.525 0.52916667 0.53333333 0.5375 0.54166667 0.54583333 0.55 0.55416667 0.55833333 0.5625 0.56666667 0.57083333 0.575 0.57916667 0.58333333 0.5875 0.59166667 0.59583333 0.6 0.60416667 0.60833333 0.6125 0.61666667 0.62083333 0.625 0.62916667 0.63333333 0.6375 0.64166667 0.64583333 0.65 0.65416667 0.65833333 0.6625 0.66666667 0.67083333 0.675 0.67916667 0.68333333 0.6875 0.69166667 0.69583333 0.7 0.70416667 0.70833333 0.7125 0.71666667 0.72083333 0.725 0.72916667 0.73333333 0.7375 0.74166667 0.74583333 0.75 0.75416667 0.75833333 0.7625 0.76666667 0.77083333 0.775 0.77916667 0.78333333 0.7875 0.79166667 0.79583333 0.8 0.80416667 0.80833333 0.8125 0.81666667 0.82083333 0.825 0.82916667 0.83333333 0.8375 0.84166667 0.84583333 0.85 0.85416667 0.85833333 0.8625 0.86666667 0.87083333 0.875 0.87916667 0.88333333 0.8875 0.89166667 0.89583333 0.9 0.90416667 0.90833333 0.9125 0.91666667 0.92083333 0.925 0.92916667 0.93333333 0.9375 0.94166667 0.94583333 0.95 0.95416667 0.95833333 0.9625 0.96666667 0.97083333 0.975 0.97916667 0.98333333 0.9875 0.99166667 0.99583333 1 1 1 1 1 1
  arc A7 (4.5335, 8.3485) -> (3.9302, 8.6489) centre (0, 0) ccw